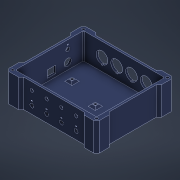
# Autodesk Inventor part: NewCase
Saved by Autodesk Inventor 2021.3 (Build 253353000, 353)
## iProperties
Created: 2021-08-09
Part Number: NewCase
Material: Generic
Document SubType Name: Modeling
Designer: Alex
Density: 1 g/cm^3
Appearance: Default
Author: Alex
Autodesk Inventor part; units mm, degrees
ref_plane "YZ Plane" through (0, 0, 0) normal (1, 0, 0) x (0, 1, 0)
ref_plane "XZ Plane" through (0, 0, 0) normal (0, 1, 0) x (-1, 0, 0)
ref_plane "XY Plane" through (0, 0, 0) normal (0, 0, 1) x (1, 0, 0)
sketch "Sketch1" plane through (0, 0, 0) normal (0, 1, 0) x (-1, 0, 0)
  line L0 (46, -55) -> (-46, -55)
  line L1 (-46, -55) -> (-50, -59)
  line L2 (-50, -59) -> (-65, -59)
  line L3 (-65, -59) -> (-69, -55)
  line L4 (-69, -55) -> (-69, -40)
  line L5 (-69, -40) -> (-65, -36)
  line L6 (-65, -36) -> (-65, 36)
  line L7 (-65, 36) -> (-69, 40)
  line L8 (-69, 40) -> (-69, 55)
  line L9 (-69, 55) -> (-65, 59)
  line L10 (-65, 59) -> (-50, 59)
  line L11 (-50, 59) -> (-46, 55)
  line L12 (-46, 55) -> (46, 55)
  line L13 (46, 55) -> (50, 59)
  line L14 (50, 59) -> (65, 59)
  line L15 (65, 59) -> (69, 55)
  line L16 (69, 55) -> (69, 40)
  line L17 (69, 40) -> (65, 36)
  line L18 (65, 36) -> (65, -36)
  line L19 (65, -36) -> (69, -40)
  line L20 (69, -40) -> (69, -55)
  line L21 (69, -55) -> (65, -59)
  line L22 (65, -59) -> (50, -59)
  line L23 (50, -59) -> (46, -55)
  point P0 (0, 0)
  point P1 (0, -55)
  point P2 (65, 0)
  dimension "d4" = 130
  dimension "d5" = 110
  dimension "d6" = 4
  dimension "d7" = 15
  dimension "d10" = 4
  dimension "d11" = 135
  dimension "d12" = 135
  constraints: 48 end point, 10 parallel, 7 equal length, 5 horizontal alignment, 4 horizontal, 4 point on line, 4 vertical, 3 collinear, 3 vertical alignment, 2 midpoint
  measures "d4" distance between parallel lines of L6 L18
  measures "d5" distance between parallel lines of L12 L0
  measures "d6" distance between parallel lines of L22 L0
  measures "d7" distance of L21.end L22.end
  measures "d10" distance between parallel lines of L4 L6
  measures "d11" angle of L12 L13
  measures "d12" angle of L11 L12
extrude "Extrusion1" add sketch "Sketch1" along normal blind 3
sketch "Sketch2" plane through (0, 3, 0) normal (0, 1, 0) x (1, 0, 0)
  line L0 (-50, 59) -> (-65, 59) projected
  line L1 (-65, 59) -> (-69, 55) projected
  line L2 (-69, 55) -> (-69, 40) projected
  line L3 (-69, 40) -> (-65, 36) projected
  line L4 (-65, 36) -> (-65, -36) projected
  line L5 (-65, -36) -> (-69, -40) projected
  line L6 (-69, -40) -> (-69, -55) projected
  line L7 (-69, -55) -> (-65, -59) projected
  line L8 (-65, -59) -> (-50, -59) projected
  line L9 (-50, -59) -> (-46, -55) projected
  line L10 (-46, -55) -> (46, -55) projected
  line L11 (46, -55) -> (50, -59) projected
  line L12 (50, -59) -> (65, -59) projected
  line L13 (65, -59) -> (69, -55) projected
  line L14 (69, -55) -> (69, -40) projected
  line L15 (69, -40) -> (65, -36) projected
  line L16 (65, -36) -> (65, 36) projected
  line L17 (65, 36) -> (69, 40) projected
  line L18 (69, 40) -> (69, 55) projected
  line L19 (69, 55) -> (65, 59) projected
  line L20 (65, 59) -> (50, 59) projected
  line L21 (50, 59) -> (46, 55) projected
  line L22 (46, 55) -> (-46, 55) projected
  line L23 (-46, 55) -> (-50, 59) projected
  line L24 (-60, 52) -> (60, 52)
  line L25 (62, 50) -> (62, -50)
  line L26 (60, -52) -> (-60, -52)
  line L27 (-62, -50) -> (-62, 50)
  line L28 (-62, 50) -> (-60, 52)
  line L29 (60, 52) -> (62, 50)
  line L30 (62, -50) -> (60, -52)
  line L31 (-60, -52) -> (-62, -50)
  point P0 (0, 0)
  point P1 (-62, 52)
  point P2 (62, -52)
  point P3 (62, 52)
  point P4 (-62, -52)
  dimension "d15" = 3
  dimension "d16" = 3
  dimension "d17" = 3
  dimension "d18" = 3
  dimension "d19" = 2
  dimension "d20" = 2
  dimension "d21" = 2
  dimension "d22" = 2
  dimension "d23" = 2
  dimension "d24" = 2
  dimension "d25" = 2
  dimension "d26" = 2
  constraints: 16 end point, 8 point on line
  measures "d15" distance between parallel lines of L22 L24
  measures "d16" distance between parallel lines of L4 L27
  measures "d17" distance between parallel lines of L10 L26
  measures "d18" distance between parallel lines of L16 L25
  measures "d19" distance of L27.end point (-62, 52)
  measures "d20" distance of L24.start point (-62, 52)
  measures "d21" distance of L24.end point (62, 52)
  measures "d22" distance of L25.start point (62, 52)
  measures "d23" distance of L25.end point (62, -52)
  measures "d24" distance of L26.start point (62, -52)
  measures "d25" distance of L26.end point (-62, -52)
  measures "d26" distance of L27.start point (-62, -52)
extrude "Extrusion2" add sketch "Sketch2" along normal blind 40
sketch "Sketch3" plane through (0, 3, 0) normal (0, 1, 0) x (1, 0, 0)
  line L0 (9.6, 18.8) -> (-59, 18.8) construction
  line L1 (-59, 18.8) -> (-59, -34.5) construction
  line L2 (-59, -34.5) -> (9.6, -34.5) construction
  line L3 (9.6, -34.5) -> (9.6, 18.8) construction
  line L4 (-60, 52) -> (-62, 50) construction
  line L5 (-62, 50) -> (-62, -50) construction
  line L6 (-62, -50) -> (-60, -52) construction
  line L7 (-60, -52) -> (60, -52) construction
  line L8 (60, -52) -> (62, -50) construction
  line L9 (62, -50) -> (62, 50) construction
  line L10 (62, 50) -> (60, 52) construction
  line L11 (60, 52) -> (-60, 52) construction
  line L12 (-46.2, 18.7) -> (-41.2, 18.7)
  line L13 (-41.2, 18.7) -> (-41.2, 13.7)
  line L14 (-41.2, 13.7) -> (-46.2, 13.7)
  line L15 (-46.2, 13.7) -> (-46.2, 18.7)
  line L16 (-46.2, 18.7) -> (-41.2, 13.7) construction
  line L17 (-41.2, 18.7) -> (-46.2, 13.7) construction
  line L18 (9.6, 3.5) -> (4.6, 3.5)
  line L19 (4.6, 3.5) -> (4.6, -1.5)
  line L20 (4.6, -1.5) -> (9.6, -1.5)
  line L21 (9.6, -1.5) -> (9.6, 3.5)
  line L22 (9.6, 3.5) -> (4.6, -1.5) construction
  line L23 (4.6, 3.5) -> (9.6, -1.5) construction
  line L24 (9.6, -24.4) -> (4.6, -24.4)
  line L25 (4.6, -24.4) -> (4.6, -29.4)
  line L26 (4.6, -29.4) -> (9.6, -29.4)
  line L27 (9.6, -29.4) -> (9.6, -24.4)
  line L28 (9.6, -24.4) -> (4.6, -29.4) construction
  line L29 (4.6, -24.4) -> (9.6, -29.4) construction
  line L30 (-47.5, -34.5) -> (-42.5, -34.5)
  line L31 (-42.5, -34.5) -> (-42.5, -29.5)
  line L32 (-42.5, -29.5) -> (-47.5, -29.5)
  line L33 (-47.5, -29.5) -> (-47.5, -34.5)
  line L34 (-47.5, -34.5) -> (-42.5, -29.5) construction
  line L35 (-42.5, -34.5) -> (-47.5, -29.5) construction
  point P0 (0, 0)
  point P1 (-43.7, 16.2)
  point P2 (-45, -32)
  point P3 (7.1, 1)
  point P4 (7.1, -26.9)
  dimension "d29" = 68.6
  dimension "d30" = 53.3
  dimension "d31" = 14
  dimension "d32" = 1.3
  dimension "d33" = 50.8
  dimension "d34" = 2.5
  dimension "d35" = 5.1
  dimension "d36" = 27.9
  dimension "d37" = 15.2
  dimension "d38" = 3
  dimension "d39" = 17.5
  dimension "d41" = 5
  constraints: 56 end point, 10 horizontal, 10 vertical, 8 midpoint, 7 equal length, 1 vertical alignment
  measures "d29" distance of L0.start L0.end
  measures "d30" distance of L2.end L0.start
  measures "d31" distance from line of point (-45, -32) L1
  measures "d32" horizontal distance of point (-43.7, 16.2) point (-45, -32)
  measures "d33" horizontal distance of point (7.1, 1) point (-43.7, 16.2)
  measures "d34" distance from line of point (-45, -32) L2
  measures "d35" vertical distance of point (7.1, -26.9) point (-45, -32)
  measures "d36" distance of point (7.1, 1) point (7.1, -26.9)
  measures "d37" vertical distance of point (-43.7, 16.2) point (7.1, 1)
  measures "d38" distance between parallel lines of L5 L1
  measures "d39" distance between parallel lines of L2 L7
  measures "d41" distance of L12.start L12.end
extrude "Extrusion3" add sketch "Sketch3" along normal blind 3
chamfer "Chamfer1" distance 3 angle 45 16 edges at (7.1, 3, -3.5) (4.6, 3, -1) (7.1, 3, 1.5) (9.6, 3, -1) (7.1, 3, 24.4) (9.6, 3, 26.9) (7.1, 3, 29.4) (4.6, 3, 26.9) (-42.5, 3, 32) (-45, 3, 29.5) (-47.5, 3, 32) (-45, 3, 34.5) (-41.2, 3, -16.2) (-43.7, 3, -13.7) (-46.2, 3, -16.2) (-43.7, 3, -18.7)
sketch "Sketch5" plane through (-62, 3, 50) normal (1, 0, 0) x (0, 0, -1)
  line L0 (68.8, 4.5) -> (15.5, 4.5) construction
  line L1 (15.5, 4.5) -> (15.5, 3) construction
  line L2 (15.5, 3) -> (68.8, 3) construction
  line L3 (68.8, 3) -> (68.8, 4.5) construction
  line L4 (59.6, 15.6) -> (47.2, 15.6)
  line L5 (47.2, 15.6) -> (47.2, 4.3)
  line L6 (47.2, 4.3) -> (59.6, 4.3)
  line L7 (59.6, 4.3) -> (59.6, 15.6)
  line L8 (68.8, 0) -> (15.5, 0) construction
  line L9 (68.7, 3) -> (63.7, 3) construction
  line L10 (63.7, 3) -> (68.7, 3) construction
  line L11 (20.5, 3) -> (15.5, 3) construction
  line L12 (15.5, 3) -> (20.5, 3) construction
  point P0 (50, -3)
  point P1 (68.8, 3.75)
  point P2 (15.5, 3.75)
  dimension "d48" = 1.5
  dimension "d49" = 12.4
  dimension "d50" = 11.3
  dimension "d51" = 0.2
  dimension "d52" = 9.2
  constraints: 16 end point, 4 vertical, 2 horizontal, 2 midpoint, 2 vertical alignment, 1 collinear
  measures "d48" distance between parallel lines of L2 L0
  measures "d49" distance of L4.start L4.end
  measures "d50" distance of L4.end L5.end
  measures "d51" distance between parallel lines of L0 L6
  measures "d52" distance between parallel lines of L3 L7
extrude "Extrusion4" cut sketch "Sketch5" against normal blind 4
sketch "Sketch6" plane through (0, 6, 0) normal (0, 1, 0) x (1, 0, 0)
  line L0 (-46.2, 13.7) -> (-41.2, 13.7) construction
  line L1 (-41.2, 13.7) -> (-41.2, 18.7) construction
  line L2 (-41.2, 18.7) -> (-46.2, 18.7) construction
  line L3 (-46.2, 18.7) -> (-46.2, 13.7) construction
  line L4 (-42.5, -34.5) -> (-42.5, -29.5) construction
  line L5 (-42.5, -29.5) -> (-47.5, -29.5) construction
  line L6 (-47.5, -29.5) -> (-47.5, -34.5) construction
  line L7 (-47.5, -34.5) -> (-42.5, -34.5) construction
  line L8 (4.6, -24.4) -> (4.6, -29.4) construction
  line L9 (4.6, -29.4) -> (9.6, -29.4) construction
  line L10 (9.6, -29.4) -> (9.6, -24.4) construction
  line L11 (9.6, -24.4) -> (4.6, -24.4) construction
  line L12 (4.6, 3.5) -> (4.6, -1.5) construction
  line L13 (4.6, -1.5) -> (9.6, -1.5) construction
  line L14 (9.6, -1.5) -> (9.6, 3.5) construction
  line L15 (9.6, 3.5) -> (4.6, 3.5) construction
  point P0 (0, 0)
  point P1 (-45, -32)
  point P2 (-43.7, 16.2)
  point P3 (7.1, 1)
  point P4 (7.1, -26.9)
  point P5 (-45, -29.5)
  point P6 (-43.7, 18.7)
  point P7 (7.1, 3.5)
  point P8 (7.1, -24.4)
  point P9 (9.6, -26.9)
  point P10 (9.6, 1)
  point P11 (-41.2, 16.2)
  point P12 (-42.5, -32)
  constraints: 8 midpoint, 4 horizontal alignment, 4 vertical alignment
hole "Hole1" at (-45, 6, 32) at (-43.7, 6, -16.2) at (7.1, 6, -1) at (7.1, 6, 26.9) direction (0, -1, 0) diameter 4 depth 5
sketch "Sketch8" plane through (0, 43, 0) normal (0, 1, 0) x (1, 0, 0)
  line L0 (-64, -54) -> (64, -54) construction
  line L1 (64, -54) -> (64, 54) construction
  line L2 (64, 54) -> (-64, 54) construction
  line L3 (-64, 54) -> (-64, -54) construction
  line L4 (-65, 59) -> (-69, 55) construction
  line L5 (-69, 55) -> (-69, 40) construction
  line L6 (-69, 40) -> (-65, 36) construction
  line L7 (-65, 36) -> (-65, -36) construction
  line L8 (-65, -36) -> (-69, -40) construction
  line L9 (-69, -40) -> (-69, -55) construction
  line L10 (-69, -55) -> (-65, -59) construction
  line L11 (-65, -59) -> (-50, -59) construction
  line L12 (-50, -59) -> (-46, -55) construction
  line L13 (-46, -55) -> (46, -55) construction
  line L14 (46, -55) -> (50, -59) construction
  line L15 (50, -59) -> (65, -59) construction
  line L16 (65, -59) -> (69, -55) construction
  line L17 (69, -55) -> (69, -40) construction
  line L18 (69, -40) -> (65, -36) construction
  line L19 (65, -36) -> (65, 36) construction
  line L20 (65, 36) -> (69, 40) construction
  line L21 (69, 40) -> (69, 55) construction
  line L22 (69, 55) -> (65, 59) construction
  line L23 (65, 59) -> (50, 59) construction
  line L24 (50, 59) -> (46, 55) construction
  line L25 (46, 55) -> (-46, 55) construction
  line L26 (-46, 55) -> (-50, 59) construction
  line L27 (-50, 59) -> (-65, 59) construction
  line L28 (-60, 52) -> (60, 52) construction
  line L29 (60, 52) -> (62, 50) construction
  line L30 (62, 50) -> (62, -50) construction
  line L31 (62, -50) -> (60, -52) construction
  line L32 (60, -52) -> (-60, -52) construction
  line L33 (-60, -52) -> (-62, -50) construction
  line L34 (-62, -50) -> (-62, 50) construction
  line L35 (-62, 50) -> (-60, 52) construction
  point P0 (0, 0)
  dimension "d69" = 1
  dimension "d70" = 1
  dimension "d71" = 1
  dimension "d72" = 1
  constraints: 8 end point, 4 coincident
  measures "d69" distance between parallel lines of L3 L7
  measures "d70" distance between parallel lines of L0 L13
  measures "d71" distance between parallel lines of L25 L2
  measures "d72" distance between parallel lines of L1 L19
hole "Hole3" at (-64, 43, 54) at (64, 43, 54) at (64, 43, -54) at (-64, 43, -54) direction (0, -1, 0) diameter 4 depth 5
sketch "Sketch9" plane through (46, 0, -55) normal (0, 0, -1) x (-1, 0, 0)
  arc A0 (13.6, 12.6018) -> (10.9, 12.6018) centre (12.25, 21.5) ccw
  arc A1 (10.9, 11.5915) -> (13.6, 11.5915) centre (12.25, 21.5) ccw
  line L0 (0, 0) -> (92, 0) construction
  line L1 (92, 0) -> (92, 43) construction
  line L2 (0, 43) -> (92, 43) construction
  line L3 (0, 0) -> (0, 43) construction
  line L4 (0, 0) -> (0, 43) construction
  line L5 (10.9, 12.6018) -> (10.9, 11.5915)
  line L6 (13.6, 12.6018) -> (13.6, 11.5915)
  line L7 (12.25, 21.5) -> (12.25, 11.5) construction
  arc A2 (13.6, 11.5915) -> (10.9, 11.5915) centre (12.25, 21.5) ccw construction
  arc A3 (36.1, 12.6018) -> (33.4, 12.6018) centre (34.75, 21.5) ccw
  arc A4 (33.4, 11.5915) -> (36.1, 11.5915) centre (34.75, 21.5) ccw
  line L8 (33.4, 12.6018) -> (33.4, 11.5915)
  line L9 (36.1, 12.6018) -> (36.1, 11.5915)
  line L10 (34.75, 21.5) -> (34.75, 11.5) construction
  arc A5 (36.1, 11.5915) -> (33.4, 11.5915) centre (34.75, 21.5) ccw construction
  arc A6 (58.6, 12.6018) -> (55.9, 12.6018) centre (57.25, 21.5) ccw
  arc A7 (55.9, 11.5915) -> (58.6, 11.5915) centre (57.25, 21.5) ccw
  line L11 (55.9, 12.6018) -> (55.9, 11.5915)
  line L12 (58.6, 12.6018) -> (58.6, 11.5915)
  line L13 (57.25, 21.5) -> (57.25, 11.5) construction
  arc A8 (58.6, 11.5915) -> (55.9, 11.5915) centre (57.25, 21.5) ccw construction
  arc A9 (81.1, 12.6018) -> (78.4, 12.6018) centre (79.75, 21.5) ccw
  arc A10 (78.4, 11.5915) -> (81.1, 11.5915) centre (79.75, 21.5) ccw
  line L14 (78.4, 12.6018) -> (78.4, 11.5915)
  line L15 (81.1, 12.6018) -> (81.1, 11.5915)
  line L16 (79.75, 21.5) -> (79.75, 11.5) construction
  arc A11 (81.1, 11.5915) -> (78.4, 11.5915) centre (79.75, 21.5) ccw construction
  line L17 (34.75, 21.5) -> (57.25, 21.5) construction
  line L18 (0, 0) -> (92, 0) projected
  point P0 (46, 0)
  point P1 (46, 0)
  point P2 (0, 21.5)
  point P3 (46, 21.5)
  point P4 (46, 0)
  dimension "d80" = 18
  dimension "d81" = 20
  dimension "d90" = 2.7
  dimension "d93" = 22.5
  constraints: 28 point on circle, 26 end point, 12 centre point, 4 coincident, 4 midpoint, 2 vertical, 1 horizontal, 1 horizontal alignment, 1 vertical alignment, 40 other
  measures "d80" diameter of A0
  measures "d81" diameter of A1
  measures "d90" distance between parallel lines of L6 L5
  measures "d93" distance of A0.centre A3.centre
extrude "Extrusion5" cut sketch "Sketch9" against normal blind 4
sketch "Sketch10" plane through (-46, 0, 55) normal (0, 0, 1) x (1, 0, 0)
  circle A0 centre (12.25, 11.5) radius 3
  arc A1 (13.25, 17.4161) -> (11.25, 17.4161) centre (12.25, 11.5) ccw
  arc A2 (13.25, 18.4282) -> (11.25, 18.4282) centre (12.25, 11.5) ccw
  line L0 (11.25, 18.4282) -> (11.25, 17.4161)
  line L1 (13.25, 18.4282) -> (13.25, 17.4161)
  line L2 (12.25, 11.5) -> (12.25, 18.5) construction
  arc A3 (11.25, 17.4161) -> (13.25, 17.4161) centre (12.25, 11.5) ccw construction
  circle A4 centre (12.25, 31.5) radius 2.5
  line L3 (0, 0) -> (92, 0) construction
  line L4 (92, 0) -> (92, 43) construction
  line L5 (0, 43) -> (92, 43) construction
  line L6 (0, 0) -> (0, 43) construction
  line L7 (0, 0) -> (0, 43) construction
  line L8 (0, 21.5) -> (92, 21.5) construction
  line L9 (92, 0) -> (92, 43) construction
  line L10 (35.75, 18.4282) -> (35.75, 17.4161)
  line L11 (33.75, 18.4282) -> (33.75, 17.4161)
  arc A5 (35.75, 18.4282) -> (33.75, 18.4282) centre (34.75, 11.5) ccw
  arc A6 (35.75, 17.4161) -> (33.75, 17.4161) centre (34.75, 11.5) ccw
  circle A7 centre (34.75, 31.5) radius 2.5
  circle A8 centre (34.75, 11.5) radius 3
  arc A9 (33.75, 17.4161) -> (35.75, 17.4161) centre (34.75, 11.5) ccw construction
  line L12 (34.75, 11.5) -> (34.75, 18.5) construction
  line L13 (58.25, 18.4282) -> (58.25, 17.4161)
  line L14 (56.25, 18.4282) -> (56.25, 17.4161)
  arc A10 (58.25, 18.4282) -> (56.25, 18.4282) centre (57.25, 11.5) ccw
  arc A11 (58.25, 17.4161) -> (56.25, 17.4161) centre (57.25, 11.5) ccw
  circle A12 centre (57.25, 31.5) radius 2.5
  circle A13 centre (57.25, 11.5) radius 3
  arc A14 (56.25, 17.4161) -> (58.25, 17.4161) centre (57.25, 11.5) ccw construction
  line L15 (57.25, 11.5) -> (57.25, 18.5) construction
  line L16 (80.75, 18.4282) -> (80.75, 17.4161)
  line L17 (78.75, 18.4282) -> (78.75, 17.4161)
  arc A15 (80.75, 18.4282) -> (78.75, 18.4282) centre (79.75, 11.5) ccw
  arc A16 (80.75, 17.4161) -> (78.75, 17.4161) centre (79.75, 11.5) ccw
  circle A17 centre (79.75, 31.5) radius 2.5
  circle A18 centre (79.75, 11.5) radius 3
  arc A19 (78.75, 17.4161) -> (80.75, 17.4161) centre (79.75, 11.5) ccw construction
  line L18 (79.75, 11.5) -> (79.75, 18.5) construction
  line L19 (92, 43) -> (0, 43) construction
  line L20 (46, 43) -> (46, 0) construction
  dimension "d101" = 6
  dimension "d102" = 12
  dimension "d104" = 1
  dimension "d105" = 1
  dimension "d106" = 5
  dimension "d107" = 20
  dimension "d108" = 10
  dimension "d111" = 22.5
  constraints: 28 end point, 28 point on circle, 20 centre point, 8 coincident, 3 midpoint, 3 vertical, 1 horizontal, 1 symmetric about line, 1 vertical alignment, 52 other
  measures "d101" diameter of A0
  measures "d102" diameter of A1
  measures "d104" distance between parallel lines of L2 L0
  measures "d105" radial gap between concentric circles of A2 A1
  measures "d106" diameter of A4
  measures "d107" distance of A0.centre A4.centre
  measures "d108" distance from line of A4.centre L8
  measures "d111" distance of L1.start L10.start
extrude "Extrusion6" cut sketch "Sketch10" against normal blind 12
sketch "Sketch11" plane through (-65, 0, -36) normal (-1, 0, 0) x (0, 0, 1)
  circle A0 centre (8, 30) radius 3
  arc A1 (9, 35.9161) -> (7, 35.9161) centre (8, 30) ccw
  arc A2 (9, 36.9282) -> (7, 36.9282) centre (8, 30) ccw
  line L0 (7, 36.9282) -> (7, 35.9161)
  line L1 (9, 36.9282) -> (9, 35.9161)
  line L2 (8, 30) -> (8, 37) construction
  arc A3 (7, 35.9161) -> (9, 35.9161) centre (8, 30) ccw construction
  circle A4 centre (8, 13) radius 5.5
  line L3 (38.8, 7.3) -> (26.4, 7.3) construction
  line L4 (26.4, 7.3) -> (26.4, 18.6) construction
  line L5 (26.4, 18.6) -> (38.8, 18.6) construction
  line L6 (38.8, 18.6) -> (38.8, 7.3) construction
  line L7 (0, 0) -> (72, 0) construction
  line L8 (72, 0) -> (72, 43) construction
  line L9 (0, 43) -> (72, 43) construction
  line L10 (0, 0) -> (0, 43) construction
  line L11 (0, 0) -> (0, 43) construction
  line L12 (0, 21.5) -> (72, 21.5) construction
  line L13 (72, 0) -> (72, 43) construction
  point P0 (36, 0)
  dimension "d118" = 6
  dimension "d119" = 12
  dimension "d120" = 1
  dimension "d121" = 1
  dimension "d122" = 11
  dimension "d123" = 8.5
  dimension "d124" = 8.5
  dimension "d125" = 8
  constraints: 8 end point, 7 point on circle, 5 centre point, 3 vertical, 2 coincident, 2 midpoint, 1 vertical alignment, 1 other
  measures "d118" diameter of A0
  measures "d119" diameter of A1
  measures "d120" distance between parallel lines of L2 L0
  measures "d121" radial gap between concentric circles of A2 A1
  measures "d122" diameter of A4
  measures "d123" distance from line of L12 A0.centre
  measures "d124" distance from line of L12 A4.centre
  measures "d125" distance from line of L10 A0.centre
extrude "Extrusion7" cut sketch "Sketch11" against normal blind 12
sketch "Sketch12" plane through (-65, 0, -36) normal (-1, 0, 0) x (0, 0, 1)
  line L0 (18, 37.5) -> (28, 37.5) construction
  line L1 (28, 37.5) -> (28, 22.5) construction
  line L2 (28, 22.5) -> (18, 22.5) construction
  line L3 (18, 22.5) -> (18, 37.5) construction
  circle A0 centre (8, 13) radius 5.5 construction
  arc A1 (9, 35.9161) -> (7, 35.9161) centre (8, 30) ccw construction
  line L4 (7, 35.9161) -> (7, 36.9282) construction
  arc A2 (9, 36.9282) -> (7, 36.9282) centre (8, 30) ccw construction
  line L5 (9, 36.9282) -> (9, 35.9161) construction
  circle A3 centre (8, 30) radius 3 construction
  line L6 (38.8, 7.3) -> (26.4, 7.3) construction
  line L7 (26.4, 7.3) -> (26.4, 18.6) construction
  line L8 (26.4, 18.6) -> (38.8, 18.6) construction
  line L9 (38.8, 18.6) -> (38.8, 7.3) construction
  line L10 (0, 0) -> (72, 0) construction
  line L11 (72, 0) -> (72, 43) construction
  line L12 (0, 43) -> (72, 43) construction
  line L13 (0, 0) -> (0, 43) construction
  line L14 (20.783, 33.3056) -> (18.6549, 33.3056)
  line L15 (18.6549, 33.3056) -> (18.6549, 36.588)
  spline S0 degree 2 poles (18.6549, 36.588) (18.6549, 36.7499) (18.8114, 36.7499) knots 0 0 0 1 1 1
  spline S1 degree 2 poles (18.8114, 36.7499) (18.9653, 36.7499) (18.9653, 36.588) knots 0 0 0 1 1 1
  line L16 (18.9653, 36.588) -> (18.9653, 33.6213)
  line L17 (18.9653, 33.6213) -> (20.783, 33.6213)
  spline S2 degree 2 poles (20.783, 33.6213) (20.9395, 33.6213) (20.9395, 33.4648) knots 0 0 0 1 1 1
  spline S3 degree 2 poles (20.9395, 33.4648) (20.9395, 33.3056) (20.783, 33.3056) knots 0 0 0 1 1 1
  spline S4 degree 2 poles (24.1556, 34.9906) (24.1556, 34.2794) (23.8213, 33.7832) knots 0 0 0 1 1 1
  spline S5 degree 2 poles (23.8213, 33.7832) (23.4551, 33.2392) (22.8607, 33.2392) knots 0 0 0 1 1 1
  spline S6 degree 2 poles (22.8607, 33.2392) (22.2716, 33.2392) (21.8948, 33.7832) knots 0 0 0 1 1 1
  spline S7 degree 2 poles (21.8948, 33.7832) (21.5445, 34.29) (21.5445, 34.9906) knots 0 0 0 1 1 1
  spline S8 degree 2 poles (21.5445, 34.9906) (21.5445, 35.6964) (21.8736, 36.2165) knots 0 0 0 1 1 1
  spline S9 degree 2 poles (21.8736, 36.2165) (22.2345, 36.779) (22.805, 36.779) knots 0 0 0 1 1 1
  spline S10 degree 2 poles (22.805, 36.779) (23.4153, 36.779) (23.8, 36.2165) knots 0 0 0 1 1 1
  spline S11 degree 2 poles (23.8, 36.2165) (24.1556, 35.6964) (24.1556, 34.9906) knots 0 0 0 1 1 1
  spline S12 degree 2 poles (23.8451, 34.9906) (23.8451, 35.5796) (23.5851, 35.9909) knots 0 0 0 1 1 1
  spline S13 degree 2 poles (23.5851, 35.9909) (23.2959, 36.458) (22.805, 36.458) knots 0 0 0 1 1 1
  spline S14 degree 2 poles (22.805, 36.458) (22.3486, 36.458) (22.0885, 35.9909) knots 0 0 0 1 1 1
  spline S15 degree 2 poles (22.0885, 35.9909) (21.8603, 35.585) (21.8603, 34.9906) knots 0 0 0 1 1 1
  spline S16 degree 2 poles (21.8603, 34.9906) (21.8603, 34.4068) (22.1097, 34.0008) knots 0 0 0 1 1 1
  spline S17 degree 2 poles (22.1097, 34.0008) (22.3884, 33.555) (22.8607, 33.555) knots 0 0 0 1 1 1
  spline S18 degree 2 poles (22.8607, 33.555) (23.3383, 33.555) (23.6063, 34.0008) knots 0 0 0 1 1 1
  spline S19 degree 2 poles (23.6063, 34.0008) (23.8451, 34.4015) (23.8451, 34.9906) knots 0 0 0 1 1 1
  spline S20 degree 2 poles (27.1647, 33.7885) (26.9126, 33.4781) (26.6579, 33.356) knots 0 0 0 1 1 1
  spline S21 degree 2 poles (26.6579, 33.356) (26.4244, 33.2392) (26.0847, 33.2392) knots 0 0 0 1 1 1
  spline S22 degree 2 poles (26.0847, 33.2392) (25.5089, 33.2392) (24.758, 34.2237) (24.758, 35.041) knots 0 0 0 1 2 2 2
  spline S23 degree 2 poles (24.758, 35.041) (24.758, 35.9352) (25.1852, 36.4022) knots 0 0 0 1 1 1
  spline S24 degree 2 poles (25.1852, 36.4022) (25.5248, 36.779) (26.0078, 36.779) knots 0 0 0 1 1 1
  spline S25 degree 2 poles (26.0078, 36.779) (26.3925, 36.779) (26.6075, 36.6729) knots 0 0 0 1 1 1
  spline S26 degree 2 poles (26.6075, 36.6729) (26.8463, 36.5508) (27.0241, 36.2404) knots 0 0 0 1 1 1
  spline S27 degree 2 poles (27.0241, 36.2404) (27.048, 36.2006) (27.048, 36.1608) knots 0 0 0 1 1 1
  spline S28 degree 2 poles (27.048, 36.1608) (27.048, 36.0997) (26.9524, 36.0069) (26.8861, 36.0069) knots 0 0 0 1 2 2 2
  spline S29 degree 2 poles (26.8861, 36.0069) (26.8038, 36.0069) (26.7587, 36.0891) knots 0 0 0 1 1 1
  spline S30 degree 2 poles (26.7587, 36.0891) (26.6313, 36.3014) (26.4483, 36.3863) knots 0 0 0 1 1 1
  spline S31 degree 2 poles (26.4483, 36.3863) (26.2917, 36.458) (26.0078, 36.458) knots 0 0 0 1 1 1
  spline S32 degree 2 poles (26.0078, 36.458) (25.631, 36.458) (25.3789, 36.1422) knots 0 0 0 1 1 1
  spline S33 degree 2 poles (25.3789, 36.1422) (25.0684, 35.7627) (25.0684, 35.041) knots 0 0 0 1 1 1
  spline S34 degree 2 poles (25.0684, 35.041) (25.0684, 34.3882) (25.6522, 33.555) (26.0953, 33.555) knots 0 0 0 1 2 2 2
  spline S35 degree 2 poles (26.0953, 33.555) (26.5756, 33.555) (26.9312, 33.9902) knots 0 0 0 1 1 1
  spline S36 degree 2 poles (26.9312, 33.9902) (26.9763, 34.0459) (27.0426, 34.0459) knots 0 0 0 1 1 1
  spline S37 degree 2 poles (27.0426, 34.0459) (27.1037, 34.0459) (27.2019, 33.9504) (27.2019, 33.8894) knots 0 0 0 1 2 2 2
  spline S38 degree 2 poles (27.2019, 33.8894) (27.2019, 33.8336) (27.1647, 33.7885) knots 0 0 0 1 1 1
  spline S39 degree 2 poles (20.8613, 25.7285) (20.8613, 25.2164) (20.5269, 24.9617) knots 0 0 0 1 1 1
  spline S40 degree 2 poles (20.5269, 24.9617) (20.2961, 24.7892) (20.0785, 24.7892) knots 0 0 0 1 1 1
  line L18 (20.0785, 24.7892) -> (19.9007, 24.7892)
  line L19 (19.9007, 24.7892) -> (20.8321, 23.4784)
  spline S41 degree 2 poles (20.8321, 23.4784) (20.8613, 23.4332) (20.8613, 23.3828) knots 0 0 0 1 1 1
  spline S42 degree 2 poles (20.8613, 23.3828) (20.8613, 23.3218) (20.7657, 23.2263) (20.7047, 23.2263) knots 0 0 0 1 2 2 2
  spline S43 degree 2 poles (20.7047, 23.2263) (20.6277, 23.2263) (20.5826, 23.2926) knots 0 0 0 1 1 1
  line L20 (20.5826, 23.2926) -> (19.5106, 24.7892)
  line L21 (19.5106, 24.7892) -> (18.7199, 24.7892)
  line L22 (18.7199, 24.7892) -> (18.7199, 23.3881)
  spline S44 degree 2 poles (18.7199, 23.3881) (18.7199, 23.2263) (18.5633, 23.2263) knots 0 0 0 1 1 1
  spline S45 degree 2 poles (18.5633, 23.2263) (18.4041, 23.2263) (18.4041, 23.3881) knots 0 0 0 1 1 1
  line L23 (18.4041, 23.3881) -> (18.4041, 26.705)
  line L24 (18.4041, 26.705) -> (19.8874, 26.705)
  spline S46 degree 2 poles (19.8874, 26.705) (20.2828, 26.705) (20.5614, 26.4503) knots 0 0 0 1 1 1
  spline S47 degree 2 poles (20.5614, 26.4503) (20.8613, 26.177) (20.8613, 25.7285) knots 0 0 0 1 1 1
  spline S48 degree 2 poles (20.5508, 25.7285) (20.5508, 26.0337) (20.3491, 26.2221) knots 0 0 0 1 1 1
  spline S49 degree 2 poles (20.3491, 26.2221) (20.1607, 26.3893) (19.8874, 26.3893) knots 0 0 0 1 1 1
  line L25 (19.8874, 26.3893) -> (18.7199, 26.3893)
  line L26 (18.7199, 26.3893) -> (18.7199, 25.1103)
  line L27 (18.7199, 25.1103) -> (20.0785, 25.1103)
  spline S50 degree 2 poles (20.0785, 25.1103) (20.2111, 25.1103) (20.3518, 25.2323) knots 0 0 0 1 1 1
  spline S51 degree 2 poles (20.3518, 25.2323) (20.5508, 25.3995) (20.5508, 25.7285) knots 0 0 0 1 1 1
  line L28 (23.6209, 23.2714) -> (21.4928, 23.2714)
  line L29 (21.4928, 23.2714) -> (21.4928, 26.7103)
  line L30 (21.4928, 26.7103) -> (23.6209, 26.7103)
  spline S52 degree 2 poles (23.6209, 26.7103) (23.7775, 26.7103) (23.7775, 26.5511) knots 0 0 0 1 1 1
  spline S53 degree 2 poles (23.7775, 26.5511) (23.7775, 26.3893) (23.6209, 26.3893) knots 0 0 0 1 1 1
  line L31 (23.6209, 26.3893) -> (21.8033, 26.3893)
  line L32 (21.8033, 26.3893) -> (21.8033, 25.3172)
  line L33 (21.8033, 25.3172) -> (23.5148, 25.3172)
  spline S54 degree 2 poles (23.5148, 25.3172) (23.6766, 25.3172) (23.6766, 25.1607) knots 0 0 0 1 1 1
  spline S55 degree 2 poles (23.6766, 25.1607) (23.6766, 25.0015) (23.5148, 25.0015) knots 0 0 0 1 1 1
  line L34 (23.5148, 25.0015) -> (21.8033, 25.0015)
  line L35 (21.8033, 25.0015) -> (21.8033, 23.5871)
  line L36 (21.8033, 23.5871) -> (23.6209, 23.5871)
  spline S56 degree 2 poles (23.6209, 23.5871) (23.7775, 23.5871) (23.7775, 23.4306) knots 0 0 0 1 1 1
  spline S57 degree 2 poles (23.7775, 23.4306) (23.7775, 23.2714) (23.6209, 23.2714) knots 0 0 0 1 1 1
  spline S58 degree 2 poles (27.3438, 23.3828) (27.3438, 23.221) (27.1899, 23.221) knots 0 0 0 1 1 1
  spline S59 degree 2 poles (27.1899, 23.221) (27.0334, 23.221) (27.0334, 23.3828) knots 0 0 0 1 1 1
  line L37 (27.0334, 23.3828) -> (27.0334, 26.1558)
  line L38 (27.0334, 26.1558) -> (26.1205, 24.8343)
  spline S60 degree 2 poles (26.1205, 24.8343) (26.0383, 24.7175) (25.9321, 24.7175) knots 0 0 0 1 1 1
  spline S61 degree 2 poles (25.9321, 24.7175) (25.8313, 24.7175) (25.7597, 24.821) knots 0 0 0 1 1 1
  line L39 (25.7597, 24.821) -> (24.8469, 26.1664)
  line L40 (24.8469, 26.1664) -> (24.8469, 23.3828)
  spline S62 degree 2 poles (24.8469, 23.3828) (24.8469, 23.221) (24.6903, 23.221) knots 0 0 0 1 1 1
  spline S63 degree 2 poles (24.6903, 23.221) (24.5311, 23.221) (24.5311, 23.3828) knots 0 0 0 1 1 1
  line L41 (24.5311, 23.3828) -> (24.5311, 26.5273)
  spline S64 degree 2 poles (24.5311, 26.5273) (24.5311, 26.6997) (24.7036, 26.6997) knots 0 0 0 1 1 1
  spline S65 degree 2 poles (24.7036, 26.6997) (24.8495, 26.6997) (24.9477, 26.5617) knots 0 0 0 1 1 1
  line L42 (24.9477, 26.5617) -> (25.9375, 25.1395)
  line L43 (25.9375, 25.1395) -> (26.9299, 26.5591)
  spline S66 degree 2 poles (26.9299, 26.5591) (27.044, 26.721) (27.1766, 26.721) knots 0 0 0 1 1 1
  spline S67 degree 2 poles (27.1766, 26.721) (27.3438, 26.721) (27.3438, 26.5273) knots 0 0 0 1 1 1
  line L44 (27.3438, 26.5273) -> (27.3438, 23.3828)
  point P0 (36, 0)
  point P1 (18, 30)
  dimension "d128" = 10
  dimension "d129" = 15
  dimension "d130" = 10
  constraints: 1 horizontal, 1 horizontal alignment, 1 midpoint, 2 other
  measures "d128" distance of L0.start L0.end
  measures "d129" distance of L2.end L0.start
  measures "d130" distance of point (18, 30) A1.centre
emboss "Emboss1" sketch "Sketch12" operation cut depth 1 direction (1, 0, 0)
equation "\"d10\" = d6"
equation "\"d12\" = d11"
equation "\"d16\" = d15"
equation "\"d17\" = d15"
equation "\"d18\" = d15"
equation "\"d20\" = d19"
equation "\"d21\" = d19"
equation "\"d22\" = d21"
equation "\"d23\" = d19"
equation "\"d24\" = d23"
equation "\"d25\" = d19"
equation "\"d26\" = d25"
equation "\"d70\" = d69"
equation "\"d71\" = d69"
equation "\"d72\" = d69"
equation "\"d116\" = d102"
equation "\"d126\" = d102"
body "Solid1"
